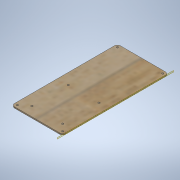
# Autodesk Inventor part: ロボット回転_回路ボード1_CPY
Saved by Autodesk Inventor 2020.3 (Build 243373000, 373)
## iProperties
Created: 2020-07-06
Part Number: ロボット回転_回路ボード1_CPY
Material: 木材 (カエデ材)
Document SubType Name: Modeling
Designer: totot
Mass: 18.3596 g
Surface Area: 285.398 cm^2
Volume: 27.4024 cm^3
Density: 0.67 g/cm^3
Appearance: ナチュラル カエデ材 - 光沢 濃い着色
Author: totot
Autodesk Inventor part; units mm, degrees
ref_plane "YZ Plane" through (0, 0, 0) normal (1, 0, 0) x (0, 1, 0)
ref_plane "XZ Plane" through (0, 0, 0) normal (0, 1, 0) x (-1, 0, 0)
ref_plane "XY Plane" through (0, 0, 0) normal (0, 0, 1) x (1, 0, 0)
sketch "スケッチ1" plane through (0, 0, 0) normal (0, 1, 0) x (-1, 0, 0)
  line L0 (0, 0) -> (-81.5097, 0)
  line L1 (-81.5097, 0) -> (-81.5097, -169)
  line L2 (-81.5097, -169) -> (0, -169)
  line L3 (0, -169) -> (0, 0)
  dimension "d0" = 169
  dimension "d7" = 81.5097
  constraints: 8 end point, 2 parallel, 1 horizontal, 1 perpendicular
  measures "d0" distance of L1.end L0.end
  measures "d7" distance between parallel lines of L1 L3
extrude "押し出し1" add sketch "スケッチ1" along normal blind 2
fillet "フィレット1" radius 4.5 4 edges at (81.5097, 1, 0) (0, 1, 0) (81.5097, 1, -169) (0, 1, -169)
sketch "スケッチ3" plane through (0, 0, 0) normal (0, -1, 0) x (1, 0, 0)
  line L0 (81.5097, -4.5) -> (81.5097, -164.5) projected
  line L1 (0, -164.5) -> (0, -4.5) projected
  line L2 (77.0097, -169) -> (4.5, -169) projected
  line L3 (4.5, 0) -> (77.0097, 0) projected
  point P0 (0, 0)
  point P1 (77.0097, -4.5)
  point P2 (77.0097, -164.5)
  point P3 (4.5, -164.5)
  point P4 (4.5, -4.5)
  dimension "d34" = 4.5
  dimension "d35" = 4.5
  dimension "d36" = 4.5
  dimension "d37" = 4.5
  dimension "d38" = 4.5
  dimension "d39" = 4.5
  dimension "d40" = 4.5
  dimension "d41" = 4.5
  measures "d34" distance from line of point (77.01, -164.5) L0
  measures "d35" distance from line of L1 point (4.5, -164.5)
  measures "d36" distance from line of point (77.01, -164.5) L2
  measures "d37" distance from line of point (4.5, -164.5) L2
  measures "d38" distance from line of L3 point (77.01, -4.5)
  measures "d39" distance from line of L3 point (4.5, -4.5)
  measures "d40" distance from line of L1 point (4.5, -4.5)
  measures "d41" distance from line of L0 point (77.01, -4.5)
hole "穴2" at (77.0097, 0, -4.5) at (77.0097, 0, -164.5) at (4.5, 0, -164.5) at (4.5, 0, -4.5) direction (0, 1, 0) diameter 3 end through all
sketch "スケッチ4" plane through (0, 0, 0) normal (0, -1, 0) x (1, 0, 0)
  line L0 (66.5097, -73) -> (17.5097, -73)
  line L1 (17.5097, -73) -> (17.5097, -15)
  line L2 (17.5097, -15) -> (66.5097, -15)
  line L3 (66.5097, -15) -> (66.5097, -73)
  line L4 (81.5097, -4.5) -> (81.5097, -164.5) projected
  line L5 (4.5, 0) -> (77.0097, 0) projected
  point P0 (0, 0)
  dimension "d49" = 49
  dimension "d50" = 58
  dimension "d51" = 15
  dimension "d52" = 15
  constraints: 8 end point, 4 coincident, 2 parallel, 1 horizontal, 1 perpendicular
  measures "d49" distance of L0.start L0.end
  measures "d50" distance of L2.end L0.start
  measures "d51" distance between parallel lines of L3 L4
  measures "d52" distance between parallel lines of L5 L2
hole "穴3" at (66.5097, 0, -73) at (17.5097, 0, -73) at (17.5097, 0, -15) at (66.5097, 0, -15) direction (0, 1, 0) diameter 3 end through all
ref_plane "作業平面1" through (81.5097, 2, 0) normal (-1, 0, 0) x (0, 0, -1)
